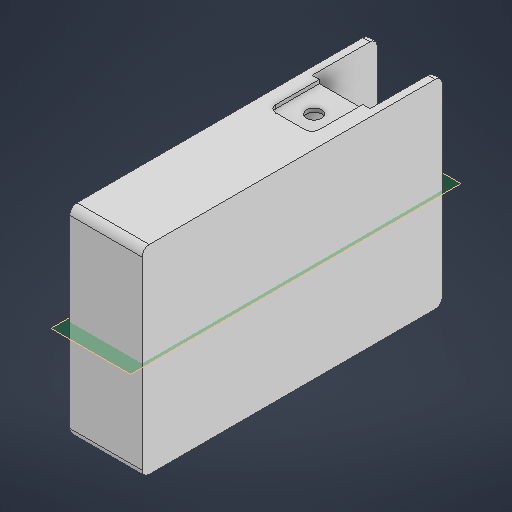
# Autodesk Inventor part: cDAQ_Chassis_LowPolyPlaceholder
Saved by Autodesk Inventor 2027 (Build 310192000, 192)
## iProperties
Created: 2026-05-14
Part Number: cDAQ_Chassis_LowPolyPlaceholder
Material: Generic
Document SubType Name: Modeling
Designer: giese
Density: 1 g/cm^3
Appearance: Default
Author: giese
Autodesk Inventor part; units mm, degrees
ref_plane "YZ Plane" through (0, 0, 0) normal (1, 0, 0) x (0, 1, 0)
ref_plane "XZ Plane" through (0, 0, 0) normal (0, 1, 0) x (-1, 0, 0)
ref_plane "XY Plane" through (0, 0, 0) normal (0, 0, 1) x (1, 0, 0)
sketch "Sketch1" plane through (0, 0, 0) normal (1, 0, 0) x (0, 1, 0)
  line L0 (55.2257, 58.6909) -> (-32.0868, 58.6909)
  line L1 (-32.0868, 58.6909) -> (-32.0868, -73.0716)
  line L2 (-32.0868, -73.0716) -> (55.2257, -73.0716)
  line L3 (55.2257, -73.0716) -> (55.2257, 58.6909)
  point P0 (0, 0)
  dimension "d0" = 131.7625
  dimension "d1" = 87.3125
  constraints: 8 end point, 2 parallel, 1 horizontal, 1 perpendicular
  measures "d0" distance between parallel lines of L2 L0
  measures "d1" distance between parallel lines of L1 L3
extrude "Extrusion1" add sketch "Sketch1" along normal blind 31.75
sketch "Sketch2" plane through (0, -32.0868, -73.0716) normal (0, -1, 0) x (1, 0, 0)
  line L0 (31.75, 131.7625) -> (31.75, 0) projected
  line L1 (0, 131.7625) -> (0, 0) projected
  line L2 (28.575, 28.575) -> (3.175, 28.575)
  line L3 (3.175, 28.575) -> (3.175, 0)
  line L4 (3.175, 0) -> (28.575, 0)
  line L5 (28.575, 0) -> (28.575, 28.575)
  point P0 (0, 73.0716)
  point P1 (31.75, 28.575)
  dimension "d7" = 3.175
  dimension "d8" = 3.175
  dimension "d9" = 28.575
  constraints: 8 end point, 2 parallel, 1 horizontal, 1 perpendicular, 1 point on line
  measures "d7" distance between parallel lines of L0 L5
  measures "d8" distance between parallel lines of L1 L3
  measures "d9" distance between parallel lines of L4 L2
extrude "Extrusion2" cut sketch "Sketch2" against normal blind 87.3125
sketch "Sketch3" plane through (28.575, -32.0868, -44.4966) normal (0, 0, -1) x (-1, 0, 0)
  line L0 (0, 0) -> (0, 87.3125) projected
  line L1 (25.4, 0) -> (25.4, 87.3125) projected
  line L2 (0, 3.175) -> (25.4, 3.175)
  line L3 (25.4, 3.175) -> (25.4, 84.1375)
  line L4 (25.4, 84.1375) -> (0, 84.1375)
  line L5 (0, 84.1375) -> (0, 3.175)
  line L6 (0, 87.3125) -> (25.4, 87.3125) projected
  line L7 (25.4, 0) -> (0, 0) projected
  point P0 (28.575, 32.0868)
  point P1 (12.7, 84.1375)
  point P2 (12.7, 3.175)
  point P3 (0, 84.1375)
  point P4 (25.4, 3.175)
  dimension "d10" = 3.175
  dimension "d11" = 3.175
  constraints: 8 end point, 2 midpoint, 2 parallel, 2 point on line, 1 horizontal, 1 perpendicular
  measures "d10" distance from line of L6 point (12.7, 84.137)
  measures "d11" distance from line of L7 point (12.7, 3.175)
extrude "Extrusion3" cut sketch "Sketch3" against normal blind 47.625 contours L0 L4 L1 L2
sketch "Sketch4" plane through (0, -32.0868, -73.0716) normal (0, -1, 0) x (1, 0, 0)
  line L0 (3.175, 28.575) -> (28.575, 28.575) projected
  line L1 (25.4, 28.575) -> (6.35, 28.575)
  line L2 (6.35, 28.575) -> (6.35, 50.8)
  line L3 (6.35, 50.8) -> (25.4, 50.8)
  line L4 (25.4, 50.8) -> (25.4, 28.575)
  line L5 (31.75, 131.7625) -> (31.75, 0) projected
  circle A0 centre (16.7802, 41.275) radius 3.302
  point P0 (0, 73.0716)
  point P1 (15.875, 50.8)
  point P2 (15.875, 28.575)
  point P3 (25.4, 39.6875)
  point P4 (6.35, 28.575)
  dimension "d14" = 22.225
  dimension "d15" = 19.05
  dimension "d16" = 6.35
  dimension "d17" = 6.604
  dimension "d18" = 12.7
  constraints: 8 end point, 3 midpoint, 2 parallel, 1 centre point, 1 horizontal, 1 perpendicular, 1 point on line
  measures "d14" distance of point (15.875, 50.8) point (15.875, 28.575)
  measures "d15" distance between parallel lines of L2 L4
  measures "d16" distance from line of L5 point (25.4, 39.687)
  measures "d17" diameter of A0
  measures "d18" distance from line of L0 A0.centre
extrude "Extrusion4" cut sketch "Sketch4" against normal blind 1.5875
sketch "Sketch6" plane through (0, -30.4993, -73.0716) normal (0, -1, 0) x (1, 0, 0)
  circle A0 centre (16.7802, 41.275) radius 3.302 projected
  circle A1 centre (16.7802, 41.275) radius 3.302
  point P0 (0, 73.0716)
  constraints: 1 centre point, 1 coincident
extrude "Extrusion5" cut sketch "Sketch6" along normal mid plane 3.175
ref_plane "Work Plane2" through (0, 11.5695, -73.0716) normal (0, -1, 0) x (1, 0, 0)
mirror "Mirror1" about plane through (0, 11.5695, -73.0716) normal (0, -1, 0) of "Extrusion4"
mirror "Mirror2" about plane through (0, 11.5695, -73.0716) normal (0, -1, 0) of "Extrusion5"
fillet "Fillet1" radius 3.175 4 edges at (30.1625, -32.0868, -73.0716) (1.5875, -32.0868, -73.0716) (30.1625, 55.2257, -73.0716) (1.5875, 55.2257, -73.0716)
fillet "Fillet2" radius 3.175 2 edges at (15.875, -32.0868, 58.6909) (15.875, 55.2257, 58.6909)
fillet "Fillet3" radius 3.175 4 edges at (6.35, -31.293, -22.2716) (25.4, -31.293, -22.2716) (25.4, 54.432, -22.2716) (6.35, 54.432, -22.2716)
body "Solid1"
